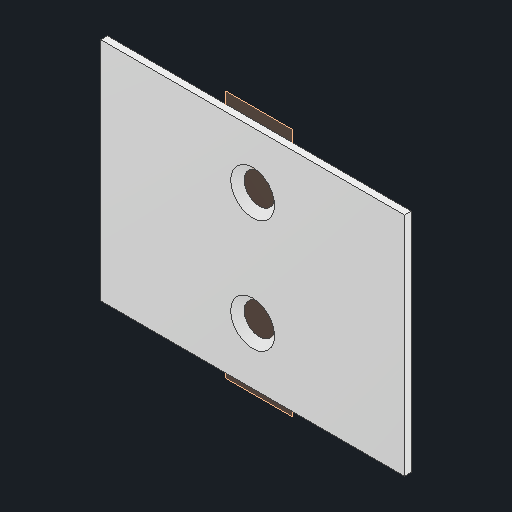
# Autodesk Inventor part: front_gear_holder
Saved by Autodesk Inventor 2023 (Build 270158000, 158)
## iProperties
Created: 2024-04-25
Part Number: front_gear_holder
Material: ABS Plastic
Document SubType Name: Modeling
Designer: szymo
Density: 1.06 g/cm^3
Appearance: Smooth - White
Mass: 1.54703 g
Surface Area: 31.227 cm^2
Volume: 1.45946 cm^3
Author: szymo
Autodesk Inventor part; units mm, degrees
ref_plane "YZ Plane" through (0, 0, 0) normal (1, 0, 0) x (0, 1, 0)
ref_plane "XZ Plane" through (0, 0, 0) normal (0, 1, 0) x (-1, 0, 0)
ref_plane "Work Plane1" through (0, 0, 0) normal (0, 0, 1) x (1, 0, 0)
sketch "Sketch1" plane through (0, 0, 0) normal (0, 0, 1) x (1, 0, 0)
  line L0 (-12, 33.5) -> (-18, 33.5) projected
  line L1 (-18, 0) -> (-18, 33.5) projected
  line L2 (-18, 0) -> (-12, 0) projected
  line L3 (27, 33.5) -> (21, 33.5) projected
  line L4 (21, 0) -> (27, 0) projected
  line L5 (27, 0) -> (27, 33.5) projected
  line L6 (-18, 33.5) -> (27, 33.5)
  line L7 (27, 33.5) -> (27, 0)
  line L8 (27, 0) -> (-18, 0)
  line L9 (-18, 0) -> (-18, 33.5)
  point P0 (0, 0)
  constraints: 8 end point, 2 parallel, 1 horizontal, 1 perpendicular
ref_plane "Work Plane2" through (-69.2, 0, 2) normal (0, 0, -1) x (0, 1, 0)
extrude "Extrusion1" add sketch "Sketch1" along normal blind 1
sketch "Sketch3" plane through (0, 0, 1) normal (0, 0, 1) x (1, 0, 0)
  circle A0 centre (4.5, 25.125) radius 2 projected
  circle A1 centre (4.5, 8.375) radius 2 projected
  point P0 (0, 0)
hole "Hole2" at (4.5, 8.375, 1) at (4.5, 25.125, 1) direction (0, 0, -1) diameter 3.6 end through all countersink diameter 6.5 countersink angle 90
body "Solid1"
